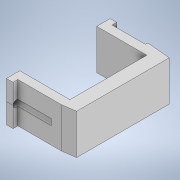
# Autodesk Inventor part: test pinza
Saved by Autodesk Inventor 2021 (Build 250183000, 183)
## iProperties
Created: 2022-04-17
Part Number: test pinza
Material: Genérico
Document SubType Name: Modeling
Designer: orgyn
Density: 1 g/cm^3
Appearance: Valor por defecto
Author: orgyn
Autodesk Inventor part; units mm, degrees
ref_plane "YZ Plane" through (0, 0, 0) normal (1, 0, 0) x (0, 1, 0)
ref_plane "XZ Plane" through (0, 0, 0) normal (0, 1, 0) x (-1, 0, 0)
ref_plane "XY Plane" through (0, 0, 0) normal (0, 0, 1) x (1, 0, 0)
sketch "Boceto1" plane through (0, 0, 0) normal (0, 1, 0) x (-1, 0, 0)
  line L0 (0, 0) -> (0, -22)
  line L1 (0, -22) -> (0, -23)
  line L2 (0, 0) -> (15, 0)
  line L3 (0, -23) -> (15, -23)
  line L4 (15, -23) -> (15, -27)
  line L5 (15, -27) -> (-4, -27)
  line L6 (-4, -27) -> (-4, 0)
  line L7 (-4, 0) -> (-4, 4)
  line L8 (-4, 4) -> (15, 4)
  line L9 (15, 4) -> (15, 0)
  line L10 (15, 4) -> (10, 4)
  line L11 (10, 4) -> (-4, 2)
  line L12 (15, -27) -> (10, -27)
  line L13 (10, -27) -> (-4, -25.6809)
  dimension "d0" = 22
  dimension "d1" = 1
  dimension "d2" = 15
  dimension "d3" = 15
  dimension "d4" = 4
  dimension "d5" = 19
  dimension "d6" = 4
  dimension "d7" = 5
  dimension "d8" = 5
  constraints: 28 end point, 5 point on line, 4 perpendicular, 2 horizontal, 2 vertical, 1 midpoint
  measures "d0" distance of L0.start L0.end
  measures "d1" distance of L0.end L1.end
  measures "d2" distance of L0.start L2.end
  measures "d3" distance of L1.end L3.end
  measures "d4" distance of L3.end L4.end
  measures "d5" distance of L4.end L5.end
  measures "d6" distance of L6.end L7.end
  measures "d7" distance of L8.end L10.end
  measures "d8" distance of L4.end L12.end
extrude "Extrusión1" add sketch "Boceto1" along normal blind 12 contours L0 L1 L3 L4 L5 L13 L6 L7 L11 L8 L9 L2
sketch "Boceto2" plane through (-15, 0, 0) normal (-1, 0, 0) x (0, 0, 1)
  line L0 (4, 0) -> (4, 12) projected
  line L1 (4, 6) -> (-27, 6)
  line L2 (-27, 0) -> (-27, 12) projected
  line L3 (4, 6) -> (3, 6)
  circle A0 centre (3, 6) radius 1
  line L4 (-27, 6) -> (-26, 6)
  circle A1 centre (-26, 6) radius 1
  point P0 (0, 0)
  dimension "d11" = 1
  dimension "d12" = 1
  constraints: 6 end point, 2 coincident, 2 horizontal alignment, 2 midpoint, 2 point on line, 4 other
  measures "d11" distance of L1.start L3.end
  measures "d12" distance of L1.end L4.end
extrude "Extrusión2" cut sketch "Boceto2" against normal blind 12
sketch "Boceto3" plane through (0, 12, 0) normal (0, 1, 0) x (1, 0, 0)
  line L0 (-10, -4) -> (4, -2) projected
  line L1 (0, -2.5714) -> (-15, -2.5714)
  line L2 (-15, -2) -> (-3, -2) projected
  line L3 (-15, -2.5714) -> (-13, -2.5714)
  line L4 (-13, -2.5714) -> (-13, -4)
  line L5 (-15, -4) -> (-10, -4) projected
  line L6 (-13, -4) -> (-10.0485, -4)
  line L7 (-10.0485, -4) -> (0, -2.5714)
  line L8 (-10, 27) -> (-15, 27) projected
  line L9 (-15, 27) -> (-13, 27)
  line L10 (-13, 27) -> (-13, 25.6179)
  line L11 (-13, 25.6179) -> (-3.0681, 25.6179)
  line L12 (-10, 27) -> (-3, 26.3405) projected
  line L13 (-3.0681, 25.6179) -> (-3, 26.3405)
  line L14 (-3, 26.3405) -> (-13, 27)
  line L15 (-13, 27) -> (-10, 27)
  line L16 (-10, 27) -> (-3, 26.3405)
  line L17 (4, 25.6809) -> (-10, 27) projected
  point P0 (0, 0)
  dimension "d15" = 2
  dimension "d16" = 2
  constraints: 24 end point, 4 perpendicular, 4 point on line, 1 collinear, 1 horizontal, 1 parallel
  measures "d15" distance of L1.end L3.end
  measures "d16" distance of L8.end L9.end
extrude "Extrusión3" cut sketch "Boceto3" against normal blind 12 contours L7 L5 L4 L1 | L12 L14 L8 | L14 L13 L11 L10
sketch "Boceto4" plane through (0, 12, 0) normal (0, 1, 0) x (1, 0, 0)
  line L0 (-10, -4) -> (0, -2.5714) projected
  line L1 (0, -2.5714) -> (-11.0485, -2.5714)
  line L2 (-15, -2) -> (-3, -2) projected
  line L3 (-11.0485, -2.5714) -> (-10.6007, -6.2769)
  line L4 (0, -2.5714) -> (4, -2) projected
  line L5 (-10.6007, -6.2769) -> (0, -2.5714)
  point P0 (0, 0)
  constraints: 6 end point, 1 parallel
extrude "Extrusión4" cut sketch "Boceto4" against normal blind 12
